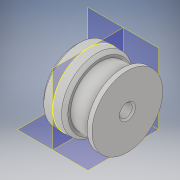
# Autodesk Inventor part: kolo1
Saved by Autodesk Inventor 2019 (Build 230136000, 136)
## iProperties
Created: 2020-05-16
Part Number: kolo1
Material: Generic
Document SubType Name: Modeling
Designer: estee
Density: 1 g/cm^3
Appearance: Default
Author: estee
Autodesk Inventor part; units mm, degrees
ref_plane "YZ Plane" through (0, 0, 0) normal (1, 0, 0) x (0, 1, 0)
ref_plane "XZ Plane" through (0, 0, 0) normal (0, 1, 0) x (-1, 0, 0)
ref_plane "XY Plane" through (0, 0, 0) normal (0, 0, 1) x (1, 0, 0)
sketch "Sketch1" plane through (0, 0, 0) normal (0, 0, 1) x (1, 0, 0)
  line L0 (0, 0) -> (0, 9.17)
  line L1 (0, 9.17) -> (-8.5, 9.17)
  line L2 (-8.5, 9.17) -> (-8.5, 11)
  line L3 (-8.5, 11) -> (-16, 11)
  line L4 (-16, 11) -> (-16, 0)
  line L5 (-16, 0) -> (0, 0)
  line L6 (0, 0) -> (0, 2)
  line L7 (0, 2) -> (-16, 2)
  line L8 (0, 9.17) -> (0, 11)
  line L9 (0, 11) -> (-1.5, 11)
  line L10 (-1.5, 11) -> (-1.5, 9.17)
  dimension "d0" = 9.17
  dimension "d1" = 8.5
  dimension "d2" = 1.83
  dimension "d3" = 7.5
  dimension "d4" = 2
  dimension "d32" = 1.5
  constraints: 22 end point, 9 perpendicular, 4 point on line, 1 vertical
  measures "d0" distance of L0.start L0.end
  measures "d1" distance of L0.end L1.end
  measures "d2" distance of L1.end L2.end
  measures "d3" distance of L2.end L3.end
  measures "d4" distance of L0.start L6.end
  measures "d32" distance of L8.end L9.end
revolve "Revolution1" add sketch "Sketch1" angle 360 about axis through (-16, 0, 0) along (1, 0, 0) contours L7 L4 L3 L2 L1 L0 | L1 L10 L9 L8
chamfer "Chamfer2" distance 1 angle 45 2 edges at (-8.5, -11, 0) (-16, -11, 0)
ref_plane "Work Plane1" through (-12.25, 0, 0) normal (-1, 0, 0) x (0, 0, 1)
sketch "Sketch3" plane through (-12.25, 0, 0) normal (-1, 0, 0) x (0, 0, 1)
  circle A0 centre (0, 0) radius 11 projected
  point P0 (0, 0)
  point P1 (-11, 0)
  constraints: 1 horizontal alignment, 1 other
ref_plane "Work Plane2" through (-12.25, 0, -11) normal (0, 0, -1) x (-1, 0, 0)
sketch "Sketch5" plane through (-12.25, 0, -11) normal (0, 0, -1) x (-1, 0, 0)
  point P0 (-12.25, 0)
  point P1 (0, 0)
hole "Hole1" at (-12.25, 0, -11) direction (0, 0, 1) diameter 3.242 depth 10 tip angle 118 thread size "M4x0.7" class "6H" standard "ISO Metric profile"
sketch "Sketch6" plane through (-12.25, 0, 0) normal (-1, 0, 0) x (0, 0, 1)
  circle A0 centre (0, 0) radius 11 projected
  point P0 (0, 0)
  point P1 (0, -11)
  constraints: 1 vertical alignment, 1 other
ref_plane "Work Plane3" through (-12.25, -11, 0) normal (0, -1, 0) x (1, 0, 0)
sketch "Sketch7" plane through (-12.25, -11, 0) normal (0, -1, 0) x (1, 0, 0)
  point P0 (12.25, 0)
  point P1 (0, 0)
hole "Hole2" at (-12.25, -11, 0) direction (0, 1, 0) diameter 3.242 depth 10 tip angle 118 thread size "M4x0.7" class "6H" standard "ISO Metric profile"
chamfer "Chamfer3" distance 0.5 angle 45 2 edges at (0, -2, 0) (-16, -2, 0)
body "Solid1"
